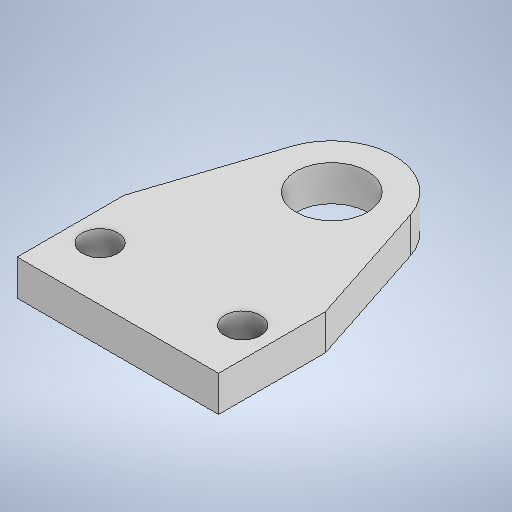
# Autodesk Inventor part: 43
Saved by Autodesk Inventor 2025.1 (Build 291241000, 241)
## iProperties
Created: 2024-09-17
Part Number: 43
Material: Generisch
Document SubType Name: Modeling
Designer: ffogue
Density: 1 g/cm^3
Appearance: Vorgabe
Author: ffogue
Autodesk Inventor part; units mm, degrees
ref_plane "YZ Plane" through (0, 0, 0) normal (1, 0, 0) x (0, 1, 0)
ref_plane "XZ Plane" through (0, 0, 0) normal (0, 1, 0) x (-1, 0, 0)
ref_plane "XY Plane" through (0, 0, 0) normal (0, 0, 1) x (1, 0, 0)
sketch "Sketch1" plane through (0, 0, 0) normal (0, 0, 1) x (1, 0, 0)
  line L0 (-5.65, 0) -> (5.65, 0)
  line L1 (5.65, 0) -> (5.65, 6)
  line L2 (5.65, 6) -> (3.3259, 13.0902)
  arc A0 (3.3259, 13.0902) -> (-3.3259, 13.0902) centre (0, 12) ccw
  line L3 (-3.3259, 13.0902) -> (-5.65, 6)
  line L4 (-5.65, 6) -> (-5.65, 0)
  line L5 (0, 0) -> (0, 14.0917) construction
  circle A1 centre (-4, 3) radius 1
  circle A2 centre (4, 3) radius 1
  circle A3 centre (0, 12) radius 2
  dimension "d0" = 3.5
  dimension "d1" = 6
  dimension "d2" = 12
  dimension "d3" = 3
  dimension "d4" = 4
  dimension "d5" = 8
  dimension "d6" = 2
  dimension "d7" = 4
  dimension "d10" = 11.3
  constraints: 12 end point, 4 centre point, 3 coincident, 3 horizontal alignment, 2 point on circle, 2 symmetric about line, 1 equal radius, 1 horizontal, 1 midpoint, 1 parallel, 1 perpendicular, 1 tangent, 1 vertical, 1 vertical alignment
  measures "d0" radius of A0
  measures "d1" distance of L3.end L0.start
  measures "d2" distance from line of L0 A0.centre
  measures "d3" distance from line of L0 A1.centre
  measures "d4" horizontal distance of point (0, 0) A1.centre
  measures "d5" distance of A2.centre A1.centre
  measures "d6" diameter of A1
  measures "d7" diameter of A3
  measures "d10" distance of L0.start L0.end
extrude "Extrusion1" add sketch "Sketch1" along normal mid plane 2
body "Solid1"
